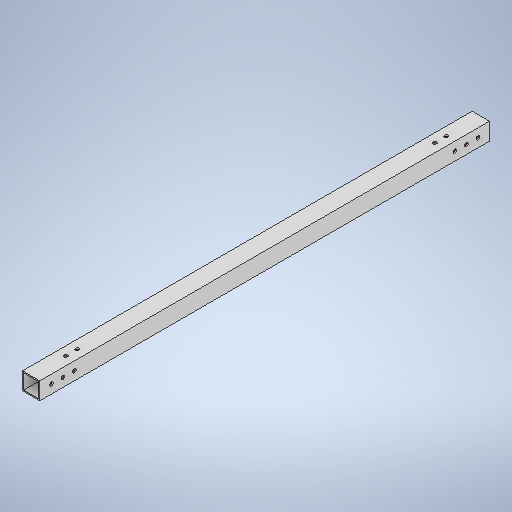
# Autodesk Inventor part: light_kaku_connect
Saved by Autodesk Inventor 2025.1 (Build 291241000, 241)
## iProperties
Created: 2025-05-06
Part Number: light_kaku_connect
Material: 一般
Document SubType Name: Modeling
Designer: yuki0520
Density: 1 g/cm^3
Appearance: 既定
Author: yuki0520
Autodesk Inventor part; units mm, degrees
ref_plane "YZ Plane" through (0, 0, 0) normal (1, 0, 0) x (0, 1, 0)
ref_plane "XZ Plane" through (0, 0, 0) normal (0, 1, 0) x (-1, 0, 0)
ref_plane "XY Plane" through (0, 0, 0) normal (0, 0, 1) x (1, 0, 0)
sketch "スケッチ1" plane through (0, 0, 0) normal (0, 0, 1) x (1, 0, 0)
  line L0 (7.5, -7.5) -> (-7.5, -7.5)
  line L1 (-7.5, -7.5) -> (-7.5, 7.5)
  line L2 (-7.5, 7.5) -> (7.5, 7.5)
  line L3 (7.5, 7.5) -> (7.5, -7.5)
  line L4 (7.5, -7.5) -> (-7.5, 7.5) construction
  line L5 (-7.5, -7.5) -> (7.5, 7.5) construction
  line L6 (6.5, 6.5) -> (-6.5, 6.5)
  line L7 (-6.5, 6.5) -> (-6.5, -6.5)
  line L8 (-6.5, -6.5) -> (6.5, -6.5)
  line L9 (6.5, -6.5) -> (6.5, 6.5)
  point P0 (0, 0)
  dimension "d0" = 15
  dimension "d1" = 15
  dimension "d2" = 1
  constraints: 20 end point, 4 parallel, 2 midpoint, 2 perpendicular, 1 horizontal, 3 other
  measures "d0" distance of L1.end L2.end
  measures "d1" distance of L0.end L1.end
  measures "d2" distance between parallel lines of L2 L6
extrude "押し出し1" add sketch "スケッチ1" along normal blind 390
sketch "スケッチ2" plane through (7.5, -7.5, 0) normal (1, 0, 0) x (0, 0, -1)
  line L0 (0, 0) -> (0, 15) projected
  line L1 (0, 15) -> (-390, 15) projected
  line L2 (-390, 0) -> (-390, 15) projected
  line L3 (0, 0) -> (-390, 0) projected
  line L4 (0, 7.5) -> (-390, 7.5)
  point P0 (-380, 7.5)
  point P1 (-370, 7.5)
  point P2 (-10, 7.5)
  point P3 (-20, 7.5)
  point P4 (-360, 7.5)
  point P5 (-30, 7.5)
  dimension "d5" = 10
  dimension "d6" = 10
  dimension "d7" = 10
  dimension "d8" = 10
  dimension "d27" = 10
  dimension "d28" = 10
  constraints: 6 point on line, 2 end point, 1 midpoint
  measures "d5" distance of point (-370, 7.5) point (-380, 7.5)
  measures "d6" distance from line of L2 point (-380, 7.5)
  measures "d7" distance of point (-10, 7.5) point (-20, 7.5)
  measures "d8" distance from line of L0 point (-10, 7.5)
  measures "d27" distance of point (-20, 7.5) point (-30, 7.5)
  measures "d28" distance of point (-370, 7.5) point (-360, 7.5)
hole "穴1" at (7.5, 0, 380) at (7.5, 0, 370) at (7.5, 0, 10) at (7.5, 0, 20) at (7.5, 0, 30) at (7.5, 0, 360) direction (-1, 0, 0) diameter 3.3 end through all
sketch "スケッチ3" plane through (-7.5, -7.5, 0) normal (0, -1, 0) x (1, 0, 0)
  line L0 (0, 0) -> (15, 0) projected
  line L1 (15, 0) -> (15, 390) projected
  line L2 (0, 390) -> (15, 390) projected
  line L3 (0, 0) -> (0, 390) projected
  line L4 (7.5, 0) -> (7.5, 390)
  point P0 (7.5, 360)
  point P1 (7.5, 350)
  point P2 (7.5, 40)
  point P3 (7.5, 30)
  dimension "d16" = 10
  dimension "d17" = 10
  dimension "d18" = 30
  dimension "d19" = 30
  constraints: 4 point on line, 2 end point, 1 midpoint
  measures "d16" distance of point (7.5, 360) point (7.5, 350)
  measures "d17" distance of point (7.5, 40) point (7.5, 30)
  measures "d18" distance from line of L0 point (7.5, 30)
  measures "d19" distance from line of L2 point (7.5, 360)
hole "穴2" at (0, -7.5, 360) at (0, -7.5, 350) at (0, -7.5, 40) at (0, -7.5, 30) direction (0, 1, 0) diameter 3.2 end through all
